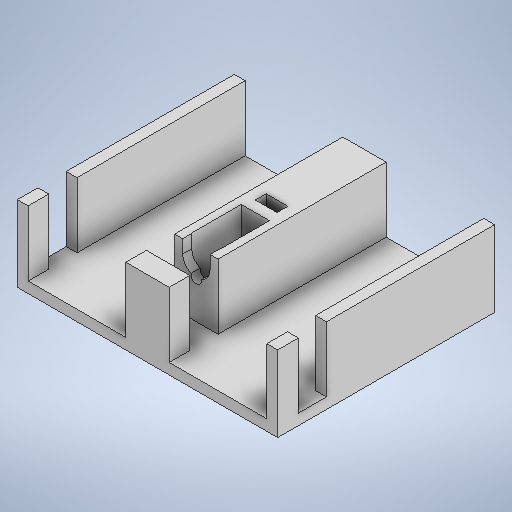
# Autodesk Inventor part: Selection Body V1
Saved by Autodesk Inventor 2025.3 (Build 293356000, 356)
## iProperties
Created: 2026-04-13
Part Number: Selection Body V1
Material: Generic
Document SubType Name: Modeling
Designer: kamal
Density: 1 g/cm^3
Appearance: Default
Author: kamal
## iProperties of the stored document Selection Body V1_3DPrint.ipt
Created: 2026-04-22
Part Number: Selection Body V1_3DPrint
Material: Generic
Document SubType Name: Modeling
Designer: kamal
Density: 1 g/cm^3
Appearance: Default
Author: kamal
Autodesk Inventor part; units mm, degrees
ref_plane "YZ Plane" through (0, 0, 0) normal (1, 0, 0) x (0, 1, 0)
ref_plane "XZ Plane" through (0, 0, 0) normal (0, 1, 0) x (-1, 0, 0)
sketch "Sketch1" plane through (0, 0, 0) normal (0, 0, 1) x (1, 0, 0)
  line L0 (0, 0) -> (0, 35) construction
  line L1 (0, 35) -> (-10, 35)
  line L2 (-10, 35) -> (-10, 5)
  line L3 (-10, 5) -> (-55, 5)
  line L4 (-55, 5) -> (-55, 35)
  line L5 (-55, 35) -> (-60, 35)
  line L6 (-60, 35) -> (-60, 0)
  line L7 (-60, 0) -> (0, 0)
  line L8 (0, 35) -> (10, 35)
  line L9 (10, 35) -> (10, 5)
  line L10 (10, 5) -> (55, 5)
  line L11 (55, 5) -> (55, 35)
  line L12 (55, 35) -> (60, 35)
  line L13 (60, 35) -> (60, 0)
  line L14 (60, 0) -> (0, 0)
  point P0 (-55, 0)
  point P1 (-10, 0)
  point P2 (55, 0)
  point P3 (10, 0)
  dimension "d0" = 35
  dimension "d1" = 10
  dimension "d2" = 30
  dimension "d3" = 45
  dimension "d4" = 5
  constraints: 30 end point, 6 perpendicular, 6 symmetric about line, 2 vertical, 1 parallel
  measures "d0" distance of L0.start L0.end
  measures "d1" distance of L0.end L1.end
  measures "d2" distance of L1.end L2.end
  measures "d3" distance of L2.end L3.end
  measures "d4" distance of L4.end L5.end
extrude "Extrusion1" add sketch "Sketch1" along normal blind 100
sketch "Sketch3" plane through (-60, 0, 0) normal (-1, 0, 0) x (0, 0, 1)
  line L0 (0, 5) -> (100, 5) projected
  line L1 (0, 35) -> (0, 0) projected
  line L2 (0, 5) -> (80, 5)
  line L3 (82.5, 5) -> (77.5, 5)
  line L4 (77.5, 5) -> (77.5, 35)
  line L5 (0, 35) -> (100, 35) projected
  line L6 (82.5, 5) -> (82.5, 35)
  point P0 (82.5, 5)
  point P1 (77.5, 5)
  dimension "d8" = 80
  dimension "d9" = 5
  constraints: 8 end point, 4 point on line, 1 midpoint, 1 parallel, 1 vertical
  measures "d8" distance of L0.start L2.end
  measures "d9" distance of L3.start L3.end
extrude "Extrusion2" cut sketch "Sketch3" against normal through all contours L4 L5 L6 L0
sketch "Sketch4" plane through (-10, 35, 0) normal (0, 1, 0) x (1, 0, 0)
  line L0 (10, 0) -> (10, -50.3)
  line L1 (16.5, -50.3) -> (3.5, -50.3)
  line L2 (3.5, -50.3) -> (3.5, -73.3)
  line L3 (3.5, -73.3) -> (16.5, -73.3)
  line L4 (16.5, -73.3) -> (16.5, -50.3)
  dimension "d12" = 50.3
  dimension "d13" = 13
  dimension "d14" = 23
  constraints: 10 end point, 2 perpendicular, 2 vertical, 1 horizontal, 1 midpoint
  measures "d12" distance of L0.start L0.end
  measures "d13" distance of L1.start L1.end
  measures "d14" distance of L1.end L2.end
extrude "Extrusion3" cut sketch "Sketch4" against normal blind 23
sketch "Sketch11" plane through (-10, 35, 77.5) normal (0, 0, 1) x (1, 0, 0)
  line L0 (20, 0) -> (0, 0) projected
  line L1 (0, 0) -> (10, 0)
  line L2 (10, 0) -> (10, -6.1) construction
  circle A0 centre (10, -6.1) radius 6.3
  line L3 (10, -6.1) -> (10, -12.4) construction
  arc A1 (12.4503, -11.904) -> (10, -9.9) centre (10, -12.4) ccw construction
  arc A2 (7.5497, -11.904) -> (12.4503, -11.904) centre (10, -12.4) ccw
  arc A3 (10, -9.9) -> (7.5497, -11.904) centre (10, -12.4) ccw construction
  line L4 (16.5, 0) -> (16.5, -23) projected
  line L5 (16.3, -6.1) -> (16.3, 0)
  line L6 (3.7, -6.1) -> (3.7, 0)
  line L7 (3.7, 0) -> (16.3, 0)
  line L8 (16.5, 0) -> (3.5, 0) projected
  point P0 (10, -35)
  point P1 (3.7, 0)
  dimension "d32" = 10
  dimension "d33" = 6.1
  dimension "d34" = 12.6
  dimension "d35" = 6.3
  dimension "d36" = 5
  constraints: 12 end point, 10 point on circle, 4 centre point, 3 point on line, 2 coincident, 2 perpendicular, 2 tangent, 1 collinear, 1 midpoint, 1 parallel, 1 vertical
  measures "d32" distance of L0.end L1.end
  measures "d33" distance of L1.end L2.end
  measures "d34" diameter of A0
  measures "d35" distance of L3.start L3.end
  measures "d36" diameter of A1
extrude "Extrusion8" cut sketch "Sketch11" against normal blind 5 contours L5 A0 L0 | A0 L0 | A0 L6 L0 | A2 A0 picked at (7.9397, -7.6935)
sketch "Sketch12" plane through (-60, 0, 0) normal (-1, 0, 0) x (0, 0, 1)
  line L0 (82.5, 35) -> (82.5, 5) projected
  line L1 (82.5, 35) -> (100, 35) projected
  line L2 (82.5, 5) -> (90.5, 5)
  line L3 (82.5, 5) -> (100, 5) projected
  line L4 (90.5, 5) -> (90.5, 35)
  point P0 (0, 0)
  dimension "d39" = 8
  constraints: 4 end point, 2 point on line, 1 perpendicular
  measures "d39" distance of L0.end L2.end
extrude "Extrusion9" cut sketch "Sketch12" against normal through all
ref_plane "Work Plane1" through (-10, 5, 84) normal (0, 0, 1) x (1, 0, 0)
sketch "Sketch14" plane through (-10, 35, 0) normal (0, 1, 0) x (1, 0, 0)
  line L0 (5, -45.3) -> (15, -45.3)
  line L1 (15, -45.3) -> (15, -40.3)
  line L2 (15, -40.3) -> (5, -40.3)
  line L3 (5, -40.3) -> (5, -45.3)
  line L4 (0, 0) -> (0, -77.5) projected
  line L5 (3.5, -50.3) -> (16.5, -50.3) projected
  point P0 (10, 0)
  point P1 (5, -42.8)
  point P2 (10, -45.3)
  point P3 (10, -50.3)
  dimension "d47" = 10
  dimension "d48" = 5
  dimension "d49" = 5
  dimension "d50" = 5
  constraints: 8 end point, 3 midpoint, 2 parallel, 1 horizontal, 1 perpendicular
  measures "d47" distance of L2.end L1.end
  measures "d48" distance of L0.end L1.end
  measures "d49" distance from line of point (5, -42.8) L4
  measures "d50" distance of point (10, -45.3) point (10, -50.3)
extrude "Extrusion11" cut sketch "Sketch14" against normal through all
equation "\"d37\" = d36"
body "Solid1"
